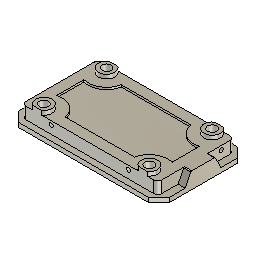
Senso Focuser top cover v2 (Autodesk Fusion 360 design; units mm, degrees)
Autodesk Fusion 360 part; units mm, degrees
sketch "Sketch1" plane through (0, 0, 0) normal (0, 0, 1) x (1, 0, 0)
  line L0 (0, 0) -> (73.72, 0)
  line L1 (73.72, 0) -> (73.72, 43.31)
  line L2 (73.72, 43.31) -> (0, 43.31)
  line L3 (0, 43.31) -> (0, 0)
  dimension "d1" = 73.72
  dimension "d2" = 43.31
  constraint horizontal L0
  constraint vertical L1
  constraint horizontal L2
  constraint vertical L3
  constraint coincident L0.start L3.end
  measures "d1" distance of L0.start L0.end
  measures "d2" distance of L0.start L2.end
extrude "Extrude1" add sketch "Sketch1" along normal blind 10
chamfer "Chamfer1" distance 5 angle 45 4 edges at (73.72, 43.31, 5) (0, 43.31, 5) (73.72, 0, 5) (0, 0, 5)
sketch "Sketch2" plane through (0, 0, 10) normal (0, 0, 1) x (-1, 0, 0)
  line L0 (0, -5) -> (-5, 0)
  line L1 (-5, 0) -> (-68.72, 0)
  line L2 (-68.72, 0) -> (-73.72, -5)
  line L3 (-73.72, -5) -> (-73.72, -38.31)
  line L4 (-73.72, -38.31) -> (-68.72, -43.31)
  line L5 (-68.72, -43.31) -> (-5, -43.31)
  line L6 (-5, -43.31) -> (0, -38.31)
  line L7 (0, -38.31) -> (0, -5)
  line L8 (0, -21.655) -> (-73.72, -21.655) construction
  line L9 (-36.86, -43.31) -> (-36.86, 0) construction
  line L10 (-5.505, -40.4) -> (-68.215, -40.4)
  line L11 (-70.215, -38.4) -> (-70.215, -4.91)
  line L12 (-68.215, -2.91) -> (-5.505, -2.91)
  line L13 (-3.505, -4.91) -> (-3.505, -38.4)
  line L14 (-3.505, -40.4) -> (-70.215, -2.91) construction
  line L15 (-70.215, -40.4) -> (-3.505, -2.91) construction
  arc A0 (-5.505, -40.4) -> (-3.505, -38.4) centre (-5.505, -38.4) ccw
  arc A1 (-70.215, -38.4) -> (-68.215, -40.4) centre (-68.215, -38.4) ccw
  arc A2 (-68.215, -2.91) -> (-70.215, -4.91) centre (-68.215, -4.91) ccw
  arc A3 (-3.505, -4.91) -> (-5.505, -2.91) centre (-5.505, -4.91) ccw
  point P0 (-36.86, -21.655)
  dimension "d6" = 37.49
  dimension "d7" = 66.71
  dimension "d8" = 2
  constraint midpoint L7 L8.start
  constraint midpoint L3 L8.end
  constraint midpoint L5 L9.start
  constraint midpoint L1 L9.end
  constraint horizontal L10
  constraint perpendicular L10 L11
  constraint parallel L10 L12
  constraint parallel L11 L13
  constraint coincident L14 P0
  constraint coincident L15 P0
  constraint midpoint L9 P0
  constraint coincident L14.start L13
  constraint coincident L14.start L10
  constraint tangent L13 A0
  constraint tangent L10 A0
  constraint coincident L15.start L10
  constraint coincident L15.start L11
  constraint tangent L10 A1
  constraint tangent L11 A1
  constraint equal A0 A1
  constraint coincident L14.end L11
  constraint coincident L14.end L12
  constraint tangent L11 A2
  constraint tangent L12 A2
  constraint equal A0 A2
  constraint coincident L15.end L12
  constraint coincident L15.end L13
  constraint tangent L12 A3
  constraint tangent L13 A3
  constraint equal A0 A3
  measures "d6" distance of L15.start L14.end
  measures "d7" distance of L14.end L15.end
  measures "d8" radius of A0
extrude "Extrude2" cut sketch "Sketch2" against normal blind 7.9
sketch "Sketch3" plane through (0, 0, 2.1) normal (0, 0, 1) x (-1, 0, 0)
  arc A0 (-5.505, -40.4) -> (-3.505, -38.4) centre (-5.505, -38.4) ccw
  line L0 (-5.505, -40.4) -> (-68.215, -40.4)
  arc A1 (-70.215, -38.4) -> (-68.215, -40.4) centre (-68.215, -38.4) ccw
  line L1 (-70.215, -38.4) -> (-70.215, -4.91)
  arc A2 (-68.215, -2.91) -> (-70.215, -4.91) centre (-68.215, -4.91) ccw
  line L2 (-68.215, -2.91) -> (-5.505, -2.91)
  arc A3 (-3.505, -4.91) -> (-5.505, -2.91) centre (-5.505, -4.91) ccw
  line L3 (-3.505, -4.91) -> (-3.505, -38.4)
  line L4 (0, -38.31) -> (0, -5)
  line L5 (0, -5) -> (-5, 0)
  line L6 (-5, 0) -> (-68.72, 0)
  line L7 (-68.72, 0) -> (-73.72, -5)
  line L8 (-73.72, -5) -> (-73.72, -38.31)
  line L9 (-73.72, -38.31) -> (-68.72, -43.31)
  line L10 (-68.72, -43.31) -> (-5, -43.31)
  line L11 (-5, -43.31) -> (0, -38.31)
  line L12 (-73.72, -21.655) -> (0, -21.655) construction
  line L13 (-73.72, -12.885) -> (-70.215, -12.885)
  line L14 (-73.72, -30.425) -> (-70.215, -30.425)
  dimension "d11" = 8.77
  dimension "d12" = 8.77
  constraint midpoint L8 L12.start
  constraint midpoint L4 L12.end
  constraint coincident L8 L13.start
  constraint coincident L1 L13.end
  constraint perpendicular L1 L13
  constraint coincident L8 L14.start
  constraint coincident L1 L14.end
  constraint perpendicular L1 L14
  measures "d11" distance of L12 L13
  measures "d12" distance of L12 L14
extrude "Extrude3" add sketch "Sketch3" along normal blind 5.9 contours L1 L8 L13 L14
chamfer "Chamfer2" distance 2.95 distance2 5.9 2 edges at (71.9675, 12.885, 8) (71.9675, 30.425, 8) measured on face at (71.3833, 18.7317, 8) measured on face at (71.3833, 18.7317, 8)
sketch "Sketch4" plane through (0, 0, 10) normal (0, 0, 1) x (-1, 0, 0)
  line L0 (-68.215, -40.4) -> (-5.505, -40.4)
  arc A0 (-5.505, -40.4) -> (-3.505, -38.4) centre (-5.505, -38.4) ccw
  line L1 (-3.505, -38.4) -> (-3.505, -4.91)
  arc A1 (-3.505, -4.91) -> (-5.505, -2.91) centre (-5.505, -4.91) ccw
  line L2 (-5.505, -2.91) -> (-68.215, -2.91)
  arc A2 (-68.215, -2.91) -> (-70.215, -4.91) centre (-68.215, -4.91) ccw
  line L3 (-70.215, -4.91) -> (-70.215, -38.4)
  arc A3 (-70.215, -38.4) -> (-68.215, -40.4) centre (-68.215, -38.4) ccw
  line L4 (-3.505, -21.655) -> (-70.215, -21.655) construction
  line L5 (-36.86, -40.4) -> (-36.86, -2.91) construction
  line L6 (-10.96, -37.055) -> (-62.76, -37.055) construction
  line L7 (-62.76, -37.055) -> (-62.76, -6.255) construction
  line L8 (-62.76, -6.255) -> (-10.96, -6.255) construction
  line L9 (-10.96, -6.255) -> (-10.96, -37.055) construction
  line L10 (-10.96, -37.055) -> (-62.76, -6.255) construction
  line L11 (-62.76, -37.055) -> (-10.96, -6.255) construction
  circle A4 centre (-10.96, -37.055) radius 2.25
  circle A5 centre (-62.76, -37.055) radius 2.25
  circle A6 centre (-62.76, -6.255) radius 2.25
  circle A7 centre (-10.96, -6.255) radius 2.25
  circle A8 centre (-10.96, -37.055) radius 3.345
  circle A9 centre (-62.76, -37.055) radius 3.345
  circle A10 centre (-62.76, -6.255) radius 3.345
  circle A11 centre (-10.96, -6.255) radius 3.345
  circle A12 centre (-10.96, -37.055) radius 4
  circle A13 centre (-62.76, -37.055) radius 4
  circle A14 centre (-62.76, -6.255) radius 4
  circle A15 centre (-10.96, -6.255) radius 4
  point P0 (-36.86, -21.655)
  dimension "d17" = 30.8
  dimension "d18" = 51.8
  dimension "d19" = 4.5
  dimension "d20" = 4.5
  dimension "d21" = 4.5
  dimension "d22" = 4.5
  dimension "d27" = 8
  dimension "d28" = 8
  dimension "d29" = 8
  dimension "d30" = 8
  constraint midpoint L1 L4.start
  constraint midpoint L3 L4.end
  constraint midpoint L0 L5.start
  constraint midpoint L2 L5.end
  constraint horizontal L6
  constraint perpendicular L6 L7
  constraint parallel L6 L8
  constraint parallel L7 L9
  constraint coincident L10 P0
  constraint coincident L11 P0
  constraint midpoint L5 P0
  constraint coincident L6.start L9.end
  constraint coincident L6.end L7.start
  constraint coincident L7.end L8.start
  constraint coincident L8.end L9.start
  constraint concentric A4 A8
  constraint tangent L0 A8
  constraint concentric A5 A9
  constraint tangent L0 A9
  constraint concentric A6 A10
  constraint tangent L2 A10
  constraint concentric A7 A11
  constraint tangent L2 A11
  constraint concentric A4 A12
  constraint concentric A9 A13
  constraint concentric A6 A14
  constraint concentric A11 A15
  measures "d17" distance of L6.start L8.end
  measures "d18" distance of L7.end L8.end
  measures "d19" diameter of A4
  measures "d20" diameter of A7
  measures "d21" diameter of A5
  measures "d22" diameter of A6
  measures "d27" diameter of A12
  measures "d28" diameter of A13
  measures "d29" diameter of A14
  measures "d30" diameter of A15
extrude "Extrude4" cut sketch "Sketch4" against normal blind 1 contours L0 A0 L1 A1 L2 A2 L3 A3 A12 A13 A14 A15 | L0 A13 | L0 A12 | L2 A14 | L2 A15 picked at (-64.9977, -40.0925) picked at (-13.1977, -40.0925) picked at (-64.9977, -3.2175) picked at (-13.1977, -3.2175)
extrude "Extrude5" cut sketch "Sketch4" against normal blind 6 contours A4 | A5 | A6 | A7
sketch "Sketch5" plane through (0, 2.91, 0) normal (0, -1, 0) x (1, 0, 0)
  line L0 (68.215, 9) -> (62.76, 9)
  line L1 (5.505, 9) -> (5.505, 2.1)
  line L2 (5.505, 2.1) -> (68.215, 2.1)
  line L3 (68.215, 2.1) -> (68.215, 9)
  circle A0 centre (55.86, 6.1) radius 1
  circle A1 centre (17.86, 6.1) radius 1
  line L4 (36.86, 8) -> (36.86, 2.1) construction
  line L5 (68.72, 0) -> (5, 0)
  line L6 (62.76, 9) -> (10.96, 9)
  line L7 (10.96, 9) -> (5.505, 9)
  dimension "d31" = 2
  dimension "d32" = 2
  dimension "d33" = 19
  dimension "d34" = 19
  dimension "d42" = 6.1
  constraint midpoint L2 L4.end
  measures "d31" diameter of A0
  measures "d32" diameter of A1
  measures "d33" distance of A0.centre L4
  measures "d34" distance of A1.centre L4
  measures "d42" distance of A1.centre L5
sketch "Sketch6" plane through (70.215, 0, 0) normal (1, 0, 0) x (0, 1, 0)
  line L0 (38.4, 9) -> (4.91, 9)
  line L1 (27.475, 8) -> (30.425, 2.1)
  line L2 (4.91, 2.1) -> (12.885, 2.1)
  line L3 (38.4, 2.1) -> (38.4, 9)
  circle A0 centre (34.01, 6.1) radius 1
  line L4 (43.31, 0) -> (43.31, 2.1)
  line L5 (5, 0) -> (38.31, 0)
  line L6 (4.91, 9) -> (4.91, 2.1)
  line L7 (12.885, 2.1) -> (15.835, 8)
  line L8 (15.835, 8) -> (27.475, 8)
  line L9 (30.425, 2.1) -> (38.4, 2.1)
  dimension "d35" = 2
  dimension "d36" = 9.3
  dimension "d37" = 6.1
  measures "d35" diameter of A0
  measures "d36" distance of A0.centre L4
  measures "d37" distance of A0.centre L5
sketch "Sketch7" plane through (3.505, 0, 0) normal (-1, 0, 0) x (0, -1, 0)
  line L0 (-4.91, 9) -> (-38.4, 9)
  line L1 (-38.4, 9) -> (-38.4, 2.1)
  line L2 (-38.4, 2.1) -> (-4.91, 2.1)
  line L3 (-4.91, 2.1) -> (-4.91, 9)
  circle A0 centre (-34.01, 6.1) radius 1
extrude "Extrude6" cut sketch "Sketch7" against normal blind 3.5 contours A0
extrude "Extrude7" cut sketch "Sketch6" against normal blind 3.5 contours A0
extrude "Extrude8" cut sketch "Sketch5" against normal blind 5 contours A0 | A1
extrude "Extrude9" add sketch "Sketch4" against normal blind 1 contours L0 A12 picked at (-13.1977, -40.0925)
extrude "Extrude10" add sketch "Sketch4" against normal blind 1 contours L0 A13 picked at (-64.9977, -40.0925)
extrude "Extrude11" add sketch "Sketch4" against normal blind 1 contours L2 A14 | L2 A15 picked at (-64.9977, -3.2175) picked at (-13.1977, -3.2175)
sketch "Sketch8" plane through (0, 0, 9) normal (0, 0, 1) x (-1, 0, 0)
  arc A0 (-13.1534, -2.91) -> (-8.7666, -2.91) centre (-10.96, -6.255) ccw
  line L0 (-13.1534, -2.91) -> (-60.5666, -2.91)
  arc A1 (-64.9534, -2.91) -> (-60.5666, -2.91) centre (-62.76, -6.255) ccw
  line L1 (-64.9534, -2.91) -> (-68.215, -2.91)
  arc A2 (-68.215, -2.91) -> (-70.215, -4.91) centre (-68.215, -4.91) ccw
  line L2 (-70.215, -4.91) -> (-70.215, -38.4)
  arc A3 (-70.215, -38.4) -> (-68.215, -40.4) centre (-68.215, -38.4) ccw
  line L3 (-68.215, -40.4) -> (-64.9534, -40.4)
  arc A4 (-60.5666, -40.4) -> (-64.9534, -40.4) centre (-62.76, -37.055) ccw
  line L4 (-60.5666, -40.4) -> (-13.1534, -40.4)
  arc A5 (-8.7666, -40.4) -> (-13.1534, -40.4) centre (-10.96, -37.055) ccw
  line L5 (-8.7666, -40.4) -> (-5.505, -40.4)
  arc A6 (-5.505, -40.4) -> (-3.505, -38.4) centre (-5.505, -38.4) ccw
  line L6 (-3.505, -38.4) -> (-3.505, -4.91)
  arc A7 (-3.505, -4.91) -> (-5.505, -2.91) centre (-5.505, -4.91) ccw
  line L7 (-5.505, -2.91) -> (-8.7666, -2.91)
  arc A8 (-8.505, -28.3963) -> (-19.8065, -35.4) centre (-10.96, -37.055) ccw
  line L8 (-53.9135, -35.4) -> (-19.8065, -35.4)
  arc A9 (-53.9135, -35.4) -> (-65.215, -28.3963) centre (-62.76, -37.055) ccw
  line L9 (-65.215, -14.9137) -> (-65.215, -28.3963)
  arc A10 (-65.215, -14.9137) -> (-53.9135, -7.91) centre (-62.76, -6.255) ccw
  line L10 (-19.8065, -7.91) -> (-53.9135, -7.91)
  arc A11 (-19.8065, -7.91) -> (-8.505, -14.9137) centre (-10.96, -6.255) ccw
  line L11 (-8.505, -28.3963) -> (-8.505, -14.9137)
  dimension "d51" = -5
extrude "Extrude12" cut sketch "Sketch8" against normal blind 2 contours A8 L8 A9 L9 A10 L10 A11 L11
extrude "Extrude13" add 2 faces at (72.5517, 30.425, 2.1004) (72.5517, 29.4419, 4.0675) along direction (0, 0.894427, 0.447214) blind 0.05
extrude "Extrude14" add 2 faces at (71.3833, 12.885, 2.1008) (71.3833, 14.8513, 6.0337) along direction (0, -0.894427, 0.447214) blind 0.05
ref_plane "WorkPlane1" through (71.9675, 21.655, 9) normal (0, 0, 1) x (1, 0, 0)
sketch "Sketch9" plane through (0, 0, 9) normal (0, 0, 1) x (1, 0, 0)
  line L0 (73.72, 27.5197) -> (73.72, 30.4697)
  line L1 (73.72, 30.4697) -> (70.215, 30.4697)
  line L2 (70.215, 30.4697) -> (70.215, 27.5197)
  line L3 (70.215, 27.5197) -> (73.72, 27.5197)
  line L4 (73.72, 12.8403) -> (73.72, 15.7903)
  line L5 (73.72, 15.7903) -> (70.215, 15.7903)
  line L6 (70.215, 15.7903) -> (70.215, 12.8403)
  line L7 (70.215, 12.8403) -> (73.72, 12.8403)
  line L8 (73.72, 27.475) -> (70.215, 27.475)
  line L9 (70.215, 27.475) -> (70.215, 15.835)
  line L10 (70.215, 15.835) -> (73.72, 15.835)
  line L11 (73.72, 15.835) -> (73.72, 27.475)
  line L12 (70.215, 27.475) -> (73.72, 27.475)
  line L13 (73.72, 27.475) -> (73.72, 27.5197)
  line L14 (73.72, 27.5197) -> (70.215, 27.5197)
  line L15 (70.215, 27.5197) -> (70.215, 27.475)
  line L16 (73.72, 15.835) -> (70.215, 15.835)
  line L17 (70.215, 15.835) -> (70.215, 15.7903)
  line L18 (70.215, 15.7903) -> (73.72, 15.7903)
  line L19 (73.72, 15.7903) -> (73.72, 15.835)
extrude "Extrude15" cut sketch "Sketch9" against normal blind 1
fillet "Fillet1" radius 0.5 2 edges at (71.9675, 15.7791, 8) (71.9675, 27.5309, 8)
extrude "Extrude16" add 1 faces at (2.3367, 16.1033, 2.1) along direction (0, 0, 1) blind 0.1
extrude "Extrude17" cut 1 faces at (66.715, 33.6173, 5.8733) along direction (-1, 0, 0) blind 0.5
extrude "Extrude18" cut 1 faces at (7.005, 34.4027, 5.8733) along direction (1, 0, 0) blind 1
extrude "Extrude19" cut 1 faces at (68.5483, 19.4079, 9) along direction (0, 0, -1) blind 1
equation "d11 = ( 17.54 / 2 ) * 1 mm"
equation "d12 = d11"
equation "d20 = d19"
equation "d21 = d19"
equation "d22 = d19"
